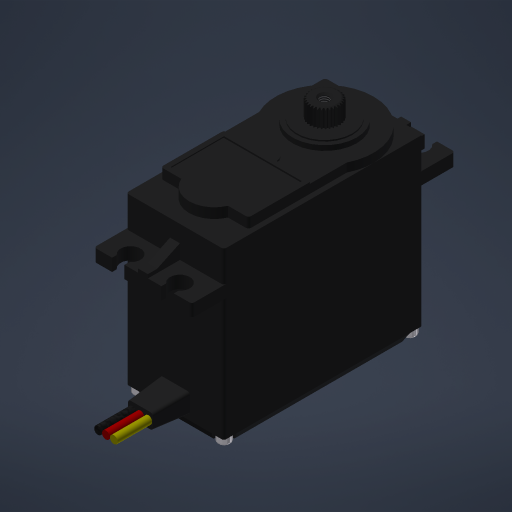
# Autodesk Inventor part: HS-645 MG
Saved by Autodesk Inventor 2023 (Build 270158000, 158)
## iProperties
Created: 2013-10-04
Part Number: HS-645 MG
Document SubType Name: Modeling
Designer: Phil
Density: 1 g/cm^3
Material: Generic
Appearance: Glossy - Black
Author: Phil
Autodesk Inventor part; units mm, degrees
ref_plane "YZ Plane" through (0, 0, 0) normal (1, 0, 0) x (0, 1, 0)
ref_plane "XZ Plane" through (0, 0, 0) normal (0, 1, 0) x (-1, 0, 0)
sketch "Sketch1" plane through (0, 0, 0) normal (0, 0, 1) x (1, 0, 0)
  line L0 (-9.9, 20.15) -> (9.9, 20.15)
  line L1 (9.9, 20.15) -> (9.9, -20.15)
  line L2 (9.9, -20.15) -> (-9.9, -20.15)
  line L3 (-9.9, -20.15) -> (-9.9, 20.15)
  point P0 (0, 0)
  dimension "d0" = 19.8
  dimension "d1" = 9.9
  dimension "d2" = 40.3
  dimension "d3" = 20.15
  constraints: 8 end point, 2 parallel, 1 horizontal, 1 perpendicular
  measures "d0" distance of L0.start L0.end
  measures "d1" distance from line of point (0, 0) L3
  measures "d2" distance between parallel lines of L2 L0
  measures "d3" distance from line of point (0, 0) L0
extrude "Extrusion1" add sketch "Sketch1" along normal blind 35.25
sketch "Sketch2" plane through (0, 0, 35.25) normal (0, 0, 1) x (1, 0, 0)
  line L0 (9.9, 20.15) -> (9.9, -20.15) projected
  line L1 (-9.9, 20.15) -> (9.9, 20.15) projected
  line L2 (0, 0) -> (0, 24.608) construction
  arc A0 (8.875, 5.7632) -> (-8.875, 5.7632) centre (0, 10.15) ccw
  line L3 (8.875, 5.7632) -> (8.875, -14.15)
  line L4 (8.875, -14.15) -> (-8.875, -14.15)
  line L5 (-8.875, -14.15) -> (-8.875, 5.7632)
  arc A1 (-4.7325, -14.15) -> (4.7325, -14.15) centre (0, -12.1834) ccw
  line L6 (-4.8, -13.0277) -> (-4.8, -17.2497) construction
  dimension "d6" = 10
  dimension "d7" = 17.75
  dimension "d8" = 8.875
  dimension "d9" = 34.3
  dimension "d10" = 4.8
  dimension "d11" = 1.9667
  dimension "d12" = 10.2498
  constraints: 10 end point, 4 point on circle, 4 point on line, 2 centre point, 2 parallel, 1 perpendicular, 1 tangent
  measures "d6" distance from line of A0.centre L1
  measures "d7" distance between parallel lines of L3 L5
  measures "d8" distance between parallel lines of L5 L2
  measures "d9" distance between parallel lines of L4 L1
  measures "d10" distance between parallel lines of L2 L6
  measures "d11" distance from line of L4 A1.centre
  measures "d12" diameter of A1
extrude "Extrusion2" add sketch "Sketch2" along normal blind 1.75
fillet "Fillet1" radius 0.5 2 edges at (8.875, -14.15, 36.125) (-8.875, -14.15, 36.125)
sketch "Sketch3" plane through (0, 0, 37) normal (0, 0, 1) x (1, 0, 0)
  arc A0 (-8.875, -13.65) -> (-8.375, -14.15) centre (-8.375, -13.65) ccw projected
  line L0 (-4.7325, -14.15) -> (-8.375, -14.15) projected
  arc A1 (-4.7325, -14.15) -> (4.7325, -14.15) centre (0, -12.1834) ccw projected
  line L1 (8.375, -14.15) -> (4.7325, -14.15) projected
  arc A2 (8.375, -14.15) -> (8.875, -13.65) centre (8.375, -13.65) ccw projected
  line L2 (8.875, 5.7632) -> (8.875, -13.65) projected
  line L3 (-8.875, -13.65) -> (-8.875, 5.7632) projected
  line L4 (-8.375, -1.35) -> (8.375, -1.35)
  line L5 (8.875, -13.65) -> (8.875, -1.85)
  line L6 (-8.875, -13.65) -> (-8.875, -1.85)
  arc A3 (-8.375, -1.35) -> (-8.875, -1.85) centre (-8.375, -1.85) ccw
  arc A4 (8.875, -1.85) -> (8.375, -1.35) centre (8.375, -1.85) ccw
  arc A5 (1.8, -1.35) -> (-1.8, -1.35) centre (0, -1.35) ccw
  line L7 (-7.875, -2.35) -> (7.875, -2.35)
  line L8 (7.875, -2.35) -> (7.875, -13.15)
  line L9 (7.875, -13.15) -> (-7.875, -13.15)
  line L10 (-7.875, -13.15) -> (-7.875, -2.35)
  point P0 (0, 0)
  point P1 (-8.875, -1.35)
  point P2 (8.875, -1.35)
  dimension "d16" = 12.8
  dimension "d17" = 0.5
  dimension "d18" = 3.6
  dimension "d19" = 1
  dimension "d20" = 1
  dimension "d21" = 1
  dimension "d22" = 1
  constraints: 14 end point, 8 point on line, 6 point on circle, 6 tangent, 3 centre point, 2 collinear, 2 parallel, 2 perpendicular, 1 equal radius, 1 horizontal, 1 midpoint
  measures "d16" distance between parallel lines of L0 L4
  measures "d17" radius of A3
  measures "d18" diameter of A5
  measures "d19" distance between parallel lines of L7 L4
  measures "d20" distance between parallel lines of L0 L9
  measures "d21" distance between parallel lines of L6 L10
  measures "d22" distance between parallel lines of L2 L8
extrude "Extrusion3" add sketch "Sketch3" along normal blind 0.3
ref_plane "Work Plane1" through (0, 0, 26.45) normal (0, 0, 1) x (1, 0, 0)
sketch "Sketch4" plane through (0, 0, 26.45) normal (0, 0, 1) x (1, 0, 0)
  line L0 (-9.9, 20.15) -> (9.9, 20.15) projected
  line L1 (9.9, -20.15) -> (-9.9, -20.15) projected
  line L2 (-9.9, -20.15) -> (9.9, -20.15)
  line L3 (9.9, -20.15) -> (9.9, -26.65)
  line L4 (-9.9, -26.65) -> (-9.9, -20.15)
  line L5 (-9.9, 20.15) -> (9.9, 20.15)
  line L6 (9.9, 20.15) -> (9.9, 26.65)
  line L7 (-9.9, 26.65) -> (-9.9, 20.15)
  line L8 (-9.9, 20.15) -> (-9.9, -20.15)
  line L9 (-9.9, 0) -> (-33.8042, 0) construction
  arc A0 (-6.25, 25.7112) -> (-3.75, 25.7112) centre (-5, 24.15) ccw
  line L10 (0, 0) -> (0, 31.9803) construction
  line L11 (-5, 24.15) -> (-5, 29.309) construction
  line L12 (-6.25, 25.7112) -> (-6.25, 26.65)
  line L13 (-3.75, 25.7112) -> (-3.75, 26.65)
  arc A1 (3.75, 25.7112) -> (6.25, 25.7112) centre (5, 24.15) ccw
  line L14 (6.25, 25.7112) -> (6.25, 26.65)
  line L15 (3.75, 25.7112) -> (3.75, 26.65)
  arc A2 (-3.75, -25.7112) -> (-6.25, -25.7112) centre (-5, -24.15) ccw
  line L16 (-6.25, -25.7112) -> (-6.25, -26.65)
  line L17 (-3.75, -25.7112) -> (-3.75, -26.65)
  arc A3 (6.25, -25.7112) -> (3.75, -25.7112) centre (5, -24.15) ccw
  line L18 (6.25, -25.7112) -> (6.25, -26.65)
  line L19 (3.75, -25.7112) -> (3.75, -26.65)
  line L20 (-6.25, 26.65) -> (-9.9, 26.65)
  line L21 (9.9, 26.65) -> (6.25, 26.65)
  line L22 (3.75, 26.65) -> (-3.75, 26.65)
  line L23 (-6.25, -26.65) -> (-9.9, -26.65)
  line L24 (9.9, -26.65) -> (6.25, -26.65)
  line L25 (3.75, -26.65) -> (-3.75, -26.65)
  dimension "d28" = 4
  dimension "d31" = 5
  dimension "d32" = 2.5
  dimension "d33" = 1.25
  dimension "d34" = 24.15
  constraints: 48 end point, 15 symmetric about line, 11 parallel, 8 point on circle, 4 centre point, 4 perpendicular, 2 horizontal, 1 collinear, 1 midpoint, 1 point on line, 3 other
  measures "d28" diameter of A0
  measures "d31" distance from line of L10 L11.start
  measures "d32" distance between parallel lines of L13 L12
  measures "d33" distance between parallel lines of L12 L11
  measures "d34" distance from line of L11.start L9
extrude "Extrusion4" add sketch "Sketch4" along normal blind 2.5
sketch "Sketch5" plane through (0, 0, 0) normal (1, 0, 0) x (0, 1, 0)
  line L0 (20.15, 28.95) -> (26.65, 28.95) projected
  line L1 (20.15, 28.95) -> (20.15, 35.25) projected
  line L2 (-20.15, 0) -> (20.15, 0) projected
  line L3 (0, 0) -> (0, 49.5083) construction
  line L4 (20.15, 28.95) -> (26.65, 28.95)
  line L5 (26.65, 28.95) -> (26.65, 29.691)
  line L6 (26.65, 29.691) -> (24.7942, 29.691)
  line L7 (24.7942, 29.691) -> (20.15, 31.866)
  line L8 (20.15, 28.95) -> (20.15, 31.866)
  dimension "d37" = 1.8558
  dimension "d38" = 0.741
  dimension "d39" = 154.905
  constraints: 12 end point, 3 perpendicular, 2 collinear, 1 point on line
  measures "d37" distance of L5.end L6.end
  measures "d38" distance between parallel lines of L0 L6
  measures "d39" angle of L6 L7
extrude "Extrusion5" add sketch "Sketch5" along normal mid plane 2
mirror "Mirror1" about plane through (0, 0, 0) normal (0, 1, 0) of "Extrusion5"
sketch "Sketch6" plane through (0, 0, 37) normal (0, 0, 1) x (1, 0, 0)
  arc A0 (8.875, 5.7632) -> (-8.875, 5.7632) centre (0, 10.15) ccw projected
  circle A1 centre (0, 10.15) radius 6.5
  point P0 (0, 0)
  dimension "d42" = 13
  constraints: 1 centre point, 1 coincident
  measures "d42" diameter of A1
extrude "Extrusion6" add sketch "Sketch6" along normal blind 1
sketch "Sketch7" plane through (0, 10.15, 38) normal (0, 0, 1) x (1, 0, 0)
  circle A0 centre (0, 0) radius 6.5 projected
  circle A1 centre (0, 0) radius 5.6
  point P0 (0, -10.15)
  dimension "d45" = 11.2
  constraints: 1 centre point, 1 coincident
  measures "d45" diameter of A1
extrude "Extrusion7" add sketch "Sketch7" along normal blind 0.26 contours A1
sketch "Sketch8" plane through (0, 10.15, 38.26) normal (0, 0, 1) x (1, 0, 0)
  circle A0 centre (0, 0) radius 5.6 projected
  circle A1 centre (0, 0) radius 2.9 construction
  line L0 (0, 0) -> (0, 7.9656)
  circle A2 centre (0, 0) radius 2.6
  point P0 (0, -10.15)
  dimension "d48" = 5.8
  dimension "d49" = 5.2
  constraints: 2 centre point, 2 coincident, 2 end point, 1 vertical
  measures "d48" diameter of A1
  measures "d49" diameter of A2
extrude "Extrusion8" add sketch "Sketch8" along normal blind 3.6 contours A2
sketch "Sketch9" plane through (0, 10.15, 38.26) normal (0, 0, 1) x (1, 0, 0)
  circle A0 centre (0, 0) radius 2.6 projected
  circle A1 centre (0, 0) radius 5.6 projected
  line L0 (0, 0) -> (0, 5.4278) construction
  line L1 (0, 3) -> (-0.1898, 2.5931)
  line L2 (0, 3) -> (0.1898, 2.5931)
  arc A2 (0.1898, 2.5931) -> (-0.1898, 2.5931) centre (0, 0) ccw
  point P0 (0, -10.15)
  point P1 (-0.1265, 2.6286)
  point P2 (0, 2.6)
  point P3 (0.1265, 2.6286)
  dimension "d52" = 0.4
  dimension "d53" = 25
  dimension "d59" = 0.1898
  dimension "d60" = 0.1898
  constraints: 6 end point, 6 point on circle, 2 point on line, 1 centre point, 1 symmetric about line, 1 vertical
  measures "d52" distance of A0.start L1.start
  measures "d53" angle of L0 L1
  measures "d59" horizontal distance of A0.start L1.end
  measures "d60" distance from line of L2.end L0
extrude "Extrusion9" add sketch "Sketch9" along normal up to surface (3.6 mm away) contours A0 L1 L2
pattern_circular "Circular Pattern1" count 30 over 360 about axis through (0, 10.15, 38.26) along (0, 0, 1) of "Extrusion9"
sketch "Sketch10" plane through (0, 10.15, 41.86) normal (0, 0, 1) x (1, 0, 0)
  arc A0 (0.8813, 2.4461) -> (0.7247, 2.4969) centre (0, 0) ccw projected
  circle A1 centre (0, 0) radius 0.95
  point P0 (0, -10.15)
  dimension "d61" = 1.9
  constraints: 1 centre point, 1 coincident
  measures "d61" diameter of A1
extrude "Extrusion10" cut sketch "Sketch10" against normal blind 3
chamfer "Chamfer1" distance 0.3 angle 45 1 edges at (-0.95, 10.15, 41.86)
thread "Thread1" size "M2x0.4" class "6H" standard "ANSI Metric M Profile" full length
sketch "Sketch11" plane through (0, 0, 0) normal (1, 0, 0) x (0, 1, 0)
  line L0 (11.4, 41.86) -> (8.9, 41.86) projected
  line L1 (11.4, 41.86) -> (12.6009, 41.86)
  line L2 (12.6009, 41.86) -> (13.4304, 41.3938)
  line L3 (13.4304, 41.3938) -> (13.4304, 42.3411)
  line L4 (13.4304, 42.3411) -> (11.4, 42.3411)
  line L5 (11.4, 42.3411) -> (11.4, 41.86)
  line L6 (10.15, 41.86) -> (10.15, 43.8631) construction
  point P0 (0, 0)
  constraints: 12 end point, 3 parallel, 1 collinear, 1 midpoint, 1 perpendicular
revolve "Revolution1" cut sketch "Sketch11" angle 360 about axis through (0, 10.15, 41.86) along (0, 0, 1)
chamfer "Chamfer2" distance 1 angle 60 4 edges at (9.9, 0, 0) (0, -20.15, 0) (-9.9, 0, 0) (0, 20.15, 0) measured on face at (-3.3, 6.7167, 0)
fillet "Fillet2" radius 0.5 12 edges at (-9.9, -20.15, 14.091) (9.9, -20.15, 14.091) (-9.9, -20.15, 32.1) (9.9, -20.15, 32.1) (-9.9, 20.15, 14.091) (-9.9, 20.15, 32.1) (9.9, 20.15, 14.091) (9.9, 20.15, 32.1) (9.9, 26.65, 27.7) (-9.9, 26.65, 27.7) (-9.9, -26.65, 27.7) (9.9, -26.65, 27.7)
sketch "Sketch12" plane through (0, 0, 0) normal (0, 0, -1) x (-1, 0, 0)
  line L0 (8.9, 19.15) -> (8.9, -19.15) projected
  circle A0 centre (8.6, 18.8) radius 1.8
  line L1 (0, 0) -> (20.712, 0) construction
  line L2 (0, 0) -> (0, -33.3743) construction
  circle A1 centre (8.6, -18.8) radius 1.8
  line L3 (-8.9, 19.15) -> (-8.9, -19.15)
  circle A2 centre (-8.6, 18.8) radius 1.8
  circle A3 centre (-8.6, -18.8) radius 1.8
  dimension "d74" = 3.6
  dimension "d75" = 8.6
  dimension "d76" = 18.8
  constraints: 6 end point, 4 centre point, 3 symmetric about line, 2 perpendicular, 3 other
  measures "d74" diameter of A0
  measures "d75" horizontal distance of L1.start A0.centre
  measures "d76" vertical distance of L1.start A0.centre
extrude "Extrusion11" cut sketch "Sketch12" against normal blind 1.7
sketch "Sketch13" plane through (0, 0, 1.7) normal (0, 0, -1) x (-1, 0, 0)
  line L0 (-9.8815, 17.536) -> (-9.8815, 19.7848) projected
  arc A0 (-9.8815, 17.536) -> (-7.3888, 20.1315) centre (-8.6, 18.8) ccw projected
  circle A1 centre (-8.6, 18.8) radius 1.2815
  point P0 (0, 0)
  constraints: 1 centre point, 1 coincident, 1 tangent
extrude "Extrusion12" add sketch "Sketch13" along normal blind 1.5
fillet "Fillet3" radius 0.5 1 edges at (9.8815, 18.8, 0.2)
sketch "Sketch14" plane through (8.6, 18.8, 0.2) normal (0, 0, -1) x (-1, 0, 0)
  circle A0 centre (0, 0) radius 0.7815 projected
  line L0 (0, 0) -> (1.475, 0) construction
  line L1 (0, 0) -> (0, -1.0052) construction
  line L2 (0.9, 0) -> (0.9, 0.2)
  line L3 (0.9, 0.2) -> (0.2, 0.2)
  line L4 (0.2, 0.2) -> (0.2, 0.9)
  line L5 (0.9, 0) -> (0.9, -0.2)
  line L6 (0.9, -0.2) -> (0.2, -0.2)
  line L7 (0.2, -0.2) -> (0.2, -0.9)
  line L8 (0.2, -0.9) -> (-0.0047, -0.9)
  line L9 (-0.9, 0) -> (-0.9, 0.2)
  line L10 (-0.9, 0.2) -> (-0.2, 0.2)
  line L11 (-0.2, 0.2) -> (-0.2, 0.9)
  line L12 (-0.9, 0) -> (-0.9, -0.2)
  line L13 (-0.9, -0.2) -> (-0.2, -0.2)
  line L14 (-0.2, -0.2) -> (-0.2, -0.9)
  line L15 (-0.2, -0.9) -> (0.0047, -0.9)
  line L16 (0.2, 0.9) -> (-0.2, 0.9)
  line L17 (0.9, 0.2) -> (-0.2, 0.2)
  line L18 (-0.2, 0.2) -> (-0.2, -0.2)
  line L19 (-0.2, -0.2) -> (0.9, -0.2)
  line L20 (0.9, -0.2) -> (0.9, 0.2)
  line L21 (-0.9, 0.2) -> (0.2, 0.2)
  line L22 (0.2, 0.2) -> (0.2, -0.2)
  line L23 (0.2, -0.2) -> (-0.9, -0.2)
  line L24 (-0.9, -0.2) -> (-0.9, 0.2)
  line L25 (0.2, 0.9) -> (-0.2, 0.9)
  line L26 (-0.2, 0.9) -> (-0.2, -0.2)
  line L27 (-0.2, -0.2) -> (0.2, -0.2)
  line L28 (0.2, -0.2) -> (0.2, 0.9)
  line L29 (0.2, -0.9) -> (-0.2, -0.9)
  line L30 (-0.2, -0.9) -> (-0.2, 0.2)
  line L31 (-0.2, 0.2) -> (0.2, 0.2)
  line L32 (0.2, 0.2) -> (0.2, -0.9)
  point P0 (8.6, -18.8)
  dimension "d82" = 0.2
  dimension "d83" = 0.2
  dimension "d85" = 0.9
  constraints: 66 end point, 11 parallel, 11 symmetric about line, 6 perpendicular, 5 horizontal, 1 point on line
  measures "d82" distance between parallel lines of L0 L3
  measures "d83" distance between parallel lines of L1 L4
  measures "d85" distance between parallel lines of L1 L2
extrude "Extrusion13" cut sketch "Sketch14" against normal blind 0.7 contours A0 L6 L22 L3 | A0 L3 L2 L5 L6 | L4 L17 L11 A0 | A0 L11 L16 L4 | L22 L19 L18 L17 | L7 L8 L15 L14 A0 | A0 L14 L19 L7 | L18 L13 A0 L10 | A0 L13 L12 L9 L10
pattern_linear "Rectangular Pattern1" count 2 spacing 17.1 along (-1, 0, 0) count 2 spacing 37.6 along (0, -1, 0) of "Extrusion12", "Fillet3", "Extrusion13"
sketch "Sketch15" plane through (-9.4, -20.15, 26.45) normal (0, -1, 0) x (1, 0, 0)
  line L0 (18.8, -24.7179) -> (0, -24.7179) projected
  line L1 (9.4, -24.7179) -> (9.4, -35.0811)
  line L2 (6.4, -23.7179) -> (12.4, -23.7179)
  line L3 (12.4, -23.7179) -> (12.4, -19.7179)
  line L4 (12.4, -19.7179) -> (6.4, -19.7179)
  line L5 (6.4, -19.7179) -> (6.4, -23.7179)
  point P0 (9.4, -26.45)
  dimension "d94" = 4
  dimension "d95" = 6
  dimension "d96" = 3
  dimension "d97" = 1
  constraints: 10 end point, 2 parallel, 2 perpendicular, 1 horizontal, 1 midpoint
  measures "d94" distance of L4.end L2.start
  measures "d95" distance between parallel lines of L3 L5
  measures "d96" distance between parallel lines of L1 L5
  measures "d97" distance between parallel lines of L0 L2
extrude "Extrusion14" add sketch "Sketch15" along normal blind 7 draft -4
fillet "Fillet4" radius 0.5 4 edges at (2.7553, -23.65, 2.9768) (-2.7553, -23.65, 2.9768) (2.7553, -23.65, 6.4873) (-2.7553, -23.65, 6.4873)
sketch "Sketch16" plane through (-9.4, -27.15, 26.45) normal (0, -1, 0) x (1, 0, 0)
  line L0 (6.8895, -22.7297) -> (6.8895, -20.7062) projected
  line L1 (11.9105, -20.7062) -> (11.9105, -22.7297) projected
  line L2 (6.8895, -21.7179) -> (11.9105, -21.7179) construction
  circle A0 centre (9.4, -21.7179) radius 0.8
  circle A1 centre (7.8, -21.7179) radius 0.8
  circle A2 centre (11, -21.7179) radius 0.8
  point P0 (9.4, -26.45)
  dimension "d101" = 1.6
  dimension "d102" = 1.6
  dimension "d103" = 1.6
  dimension "d104" = 1.6
  dimension "d105" = 1.6
  constraints: 3 centre point, 3 midpoint, 2 end point, 2 point on line
  measures "d101" diameter of A0
  measures "d102" distance of A0.centre A1.centre
  measures "d103" diameter of A1
  measures "d104" diameter of A2
  measures "d105" distance of A2.centre A0.centre
extrude "Extrusion15" add sketch "Sketch16" along normal blind 7
sketch "Sketch17" plane through (0, 0, 37) normal (0, 0, 1) x (1, 0, 0)
  line L0 (-7.875, -2.35) -> (8.3239, -2.5649) construction
  line L1 (8.3239, -2.5649) -> (8.1835, -13.15) construction
  line L2 (8.1835, -13.15) -> (-8.0154, -12.9351) construction
  line L3 (-8.0154, -12.9351) -> (-7.875, -2.35) construction
  point P0 (0, 0)
  constraints: 2 other
decal "Decal1"
sketch "Sketch18" plane through (0, 0, 37) normal (0, 0, 1) x (1, 0, 0)
  line L0 (7.875, -2.35) -> (7.875, -13.15) projected
  line L1 (-7.875, -2.35) -> (-7.875, -13.15) projected
  line L2 (7.875, -2.4617) -> (-7.875, -2.4617)
  line L3 (-7.875, -2.4617) -> (-7.875, -13.15)
  line L4 (-7.875, -13.15) -> (7.875, -13.15)
  line L5 (7.875, -13.15) -> (7.875, -2.4617)
  point P0 (0, 0)
  point P1 (-7.875, -2.4617)
  constraints: 8 end point, 2 parallel, 1 horizontal, 1 perpendicular, 1 point on line
extrude "Extrusion16" add sketch "Sketch18" along normal blind 0.1
equation "\"d1\" = 0.5 * d0"
equation "\"d3\" = 0.5 * d2"
equation "\"d8\" = 0.5 * d7"
equation "\"d20\" = d19"
equation "\"d21\" = d19"
equation "\"d22\" = d21"
equation "\"d33\" = 0.5 * d32"
equation "\"d60\" = d59"
equation "\"d83\" = d82"
equation "\"d85\" = d84"
equation "\"d96\" = 0.5 * d95"
equation "\"d102\" = d101"
equation "\"d103\" = d101"
equation "\"d104\" = d101"
equation "\"d105\" = d102"
equation "\"d84\" = 0.9"
body "Solid1"
